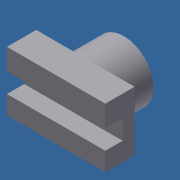
# Autodesk Inventor part: gripper
Saved by Autodesk Inventor 2012 (Build 160160000, 160)
## iProperties
Created: 2012-07-09
Part Number: gripper
Material: Aluminum-6061
Document SubType Name: Modeling
Designer: Ed
Density: 2.71 g/cm^3
Mass: 201.788 g
Surface Area: 119.758 cm^2
Volume: 74.4607 cm^3
Author: Ed
Autodesk Inventor part; units mm, degrees
ref_plane "YZ Plane" through (0, 0, 0) normal (1, 0, 0) x (0, 1, 0)
ref_plane "XZ Plane" through (0, 0, 0) normal (0, 1, 0) x (-1, 0, 0)
ref_plane "XY Plane" through (0, 0, 0) normal (0, 0, 1) x (1, 0, 0)
sketch "Sketch1" plane through (0, 0, 0) normal (0, 0, 1) x (1, 0, 0)
  circle A0 centre (0, 0) radius 19.175
  dimension "d0" = 38.35
  constraints: 1 centre point, 1 coincident
  measures "d0" diameter of A0
extrude "Extrusion1" add sketch "Sketch1" along normal blind 24.81
sketch "Sketch2" plane through (0, 0, 24.81) normal (0, 0, 1) x (1, 0, 0)
  circle A0 centre (0, 0) radius 19.175 projected
  line L0 (-31.75, 19.175) -> (31.75, 19.175)
  line L1 (31.75, 19.175) -> (31.75, -19.175)
  line L2 (31.75, -19.175) -> (-31.75, -19.175)
  line L3 (-31.75, -19.175) -> (-31.75, 19.175)
  point P0 (0, -19.175)
  dimension "d3" = 63.5
  constraints: 8 end point, 2 parallel, 2 tangent, 1 horizontal, 1 midpoint, 1 perpendicular, 1 vertical alignment
  measures "d3" distance of L0.start L0.end
extrude "Extrusion2" add sketch "Sketch2" along normal blind 18.9
sketch "Sketch3" plane through (0, 0, 0) normal (0, 0, -1) x (-1, 0, 0)
  circle A0 centre (0, 0) radius 19.175 projected
  line L0 (-15, 0) -> (15, 0)
  dimension "d6" = 30
  constraints: 2 end point, 2 horizontal alignment, 1 coincident, 1 horizontal, 1 midpoint
  measures "d6" distance of L0.start L0.end
hole "Hole1" at (15, 0, 0) at (-15, 0, 0) direction (0, 0, 1) diameter 3.302 depth 12.7 tip angle 118 thread size "8-32 UNC" class "2B" standard "ANSI Unified Screw Threads"
sketch "Sketch4" plane through (-31.75, -19.175, 24.81) normal (-1, 0, 0) x (0, 0, 1)
  line L0 (18.9, 0) -> (18.9, 38.35) projected
  line L1 (18.9, 24.7099) -> (7.724, 24.7099)
  line L2 (7.724, 24.7099) -> (7.724, 12.0099)
  line L3 (7.724, 12.0099) -> (18.9, 12.0099)
  line L4 (18.9, 12.0099) -> (18.9, 24.7099)
  point P0 (-24.81, 19.175)
  dimension "d14" = 12.7
  dimension "d15" = 11.176
  constraints: 8 end point, 2 parallel, 1 horizontal, 1 perpendicular, 1 point on line
  measures "d14" distance of L3.end L1.start
  measures "d15" distance between parallel lines of L0 L2
extrude "Extrusion3" cut sketch "Sketch4" against normal through all
body "Solid1"
